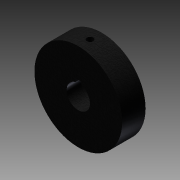
# Autodesk Inventor part: 8 ball roller plug
Saved by Autodesk Inventor 2012 (Build 160160000, 160)
## iProperties
Created: 2013-11-13
Part Number: 8 ball roller plug
Material: Default
Document SubType Name: Modeling
Designer: Bryce
Density: 1 g/cm^3
Author: Bryce
Autodesk Inventor part; units mm, degrees
ref_plane "YZ Plane" through (0, 0, 0) normal (1, 0, 0) x (0, 1, 0)
ref_plane "XZ Plane" through (0, 0, 0) normal (0, 1, 0) x (-1, 0, 0)
sketch "Sketch1" plane through (0, 0, 0) normal (0, 0, 1) x (1, 0, 0)
  circle A0 centre (0, 0) radius 23.8125
  circle A1 centre (0, 0) radius 6.35
  line L0 (-1.5875, 4.7625) -> (1.5875, 4.7625)
  line L1 (1.5875, 4.7625) -> (1.5875, 7.9375)
  line L2 (1.5875, 7.9375) -> (-1.5875, 7.9375)
  line L3 (-1.5875, 7.9375) -> (-1.5875, 4.7625)
  dimension "d0" = 47.625
  dimension "d1" = 12.7
  dimension "d2" = 3.175
  dimension "d3" = 1.5875
  dimension "d4" = 7.9375
  constraints: 8 end point, 2 centre point, 2 coincident, 2 parallel, 2 perpendicular, 1 horizontal
  measures "d0" diameter of A0
  measures "d1" diameter of A1
  measures "d2" distance of L1.end L2.end
  measures "d3" distance from line of point (0, 0) L3
  measures "d4" distance from line of point (0, 0) L2
extrude "Extrusion1" add sketch "Sketch1" along normal blind 12.7
ref_plane "Work Plane1" through (0, 23.8125, 0) normal (0, -1, 0) x (1, 0, 0)
sketch "Sketch2" plane through (0, 23.8125, 0) normal (0, -1, 0) x (1, 0, 0)
  circle A0 centre (0, 6.35) radius 1.7272
  line L0 (-23.8125, 12.7) -> (23.8125, 12.7) projected
  line L1 (-23.8125, 0) -> (23.8125, 0) projected
  line L2 (-23.8125, 0) -> (-23.8125, 12.7) projected
  line L3 (23.8125, 0) -> (23.8125, 12.7) projected
  point P0 (0, 0)
  dimension "d7" = 3.4544
  dimension "d8" = 6.35
  dimension "d9" = 23.8125
  constraints: 1 centre point
  measures "d7" diameter of A0
  measures "d8" distance from line of L1 A0.centre
  measures "d9" distance from line of L2 A0.centre
extrude "Extrusion2" cut sketch "Sketch2" along normal blind 25.4 contours A0
equation "\"d3\" = 0.5 * d2"
equation "\"d4\" = 0.5 * d1 + d3"
body "Solid1"
